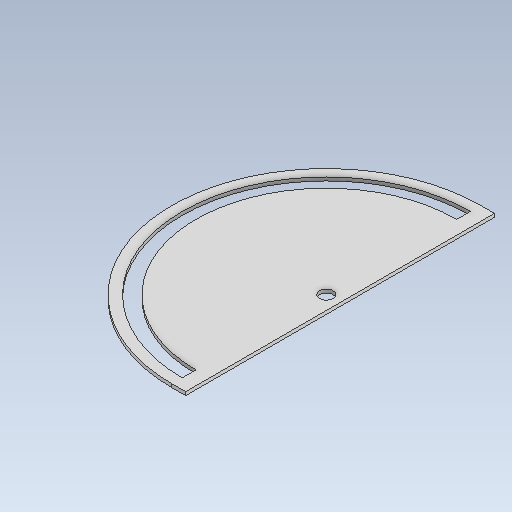
# Autodesk Inventor part: trail 12
Saved by Autodesk Inventor 2020.2 (Build 242310000, 310)
## iProperties
Created: 2020-02-19
Part Number: trail 12
Material: Generic
Document SubType Name: Modeling
Designer: lenovo
Density: 1 g/cm^3
Appearance: Default
Mass: 3.02564 g
Surface Area: 65.6255 cm^2
Volume: 3.02564 cm^3
Author: lenovo
Autodesk Inventor part; units mm, degrees
ref_plane "YZ Plane" through (0, 0, 0) normal (1, 0, 0) x (0, 1, 0)
ref_plane "XZ Plane" through (0, 0, 0) normal (0, 1, 0) x (-1, 0, 0)
ref_plane "XY Plane" through (0, 0, 0) normal (0, 0, 1) x (1, 0, 0)
sketch "Sketch1" plane through (0, 0, 0) normal (0, 1, 0) x (-1, 0, 0)
  circle A0 centre (0, 0) radius 2
  arc A1 (0, -38) -> (0, 38) centre (0, 0) ccw
  arc A2 (0, -42) -> (0, 42) centre (0, 0) ccw
  line L0 (0, 42) -> (-4, 42)
  line L1 (0, 42) -> (4, 42) construction
  line L2 (-4, 42) -> (-4, -42)
  line L3 (-4, -42) -> (0, -42)
  line L4 (0, 38) -> (0, 42)
  line L5 (0, -42) -> (0, -38)
  arc A3 (0, -45) -> (0, 45) centre (0, 0) ccw
  line L6 (0, -45) -> (-4, -45)
  line L7 (0, -45) -> (4, -45) construction
  line L8 (-4, -45) -> (-4, -42)
  line L9 (-4, 42) -> (-4, 45)
  line L10 (-4, 42) -> (-1, 42) construction
  line L11 (-4, 45) -> (0, 45)
  dimension "d0" = 4
  dimension "d1" = 76
  dimension "d2" = 38
  dimension "d3" = 84
  dimension "d4" = 4
  dimension "d5" = 180
  dimension "d6" = 84
  dimension "d7" = 90
  dimension "d8" = 45
  dimension "d9" = 4
  dimension "d10" = 180
  dimension "d11" = 3
  dimension "d12" = 90
  constraints: 24 end point, 6 point on circle, 5 horizontal, 4 centre point, 4 perpendicular, 3 equal length, 2 point on line, 1 coincident, 1 collinear, 1 concentric, 1 vertical
  measures "d0" diameter of A0
  measures "d1" distance of L5.end L4.start
  measures "d2" radius of A1
  measures "d3" distance of L3.end L0.start
  measures "d4" distance of L0.start L0.end
  measures "d5" angle of L0 L1
  measures "d6" distance of L0.end L2.end
  measures "d7" distance of L11.end L6.start
  measures "d8" radius of A3
  measures "d9" distance of L6.start L6.end
  measures "d10" angle of L6 L7
  measures "d11" distance of L0.end L9.end
  measures "d12" angle of L10 L9
extrude "Extrusion1" add sketch "Sketch1" along normal blind 1 contours L5 L3 L2 L0 L4 A1 | A2 L0 L9 L11 A3 L6 L8 L3
body "Solid1"
